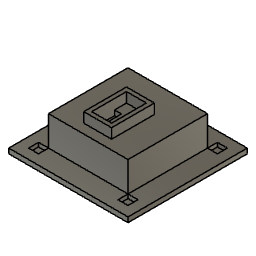
Servo Stand (Autodesk Fusion 360 design; units mm, degrees)
Autodesk Fusion 360 part; units mm, degrees
note: some values were not read from the file. Set by a fixed rule: which face or edge a step refers to.
sketch "Sketch8" plane through (0, 0, 0) normal (0, 0, 1) x (1, 0, 0)
  line L0 (10, 9.5) -> (0, 9.5)
  line L1 (-10, 9.5) -> (0, 9.5)
  line L2 (10, -27.5) -> (-10, -27.5)
  line L3 (-11, 9.5) -> (11.0117, 9.5)
  line L4 (11.0117, 9.5) -> (11.0117, -27.5)
  line L5 (11.0117, -27.5) -> (-11, -27.5)
  line L6 (-11, -27.5) -> (-11, 9.5)
  line L7 (-14, 9.5) -> (-14, 12.5)
  line L8 (-14, 12.5) -> (14, 12.5)
  line L9 (14, 12.5) -> (14, -30.5)
  line L10 (14, -30.5) -> (-14, -30.5)
  line L11 (-14, -30.5) -> (-14, 12.5)
  line L12 (0, 40) -> (-40, 40)
  line L13 (0.0067, -40) -> (40.0067, -39.9933)
  line L14 (-40, 40) -> (40.0067, 40)
  line L15 (40.0067, 40) -> (40.0067, -39.9933)
  line L16 (40.0067, -39.9933) -> (-40, -39.9933)
  line L17 (-40, -39.9933) -> (-40, 40)
  line L18 (-11, -27.5) -> (-11, -17.5)
  line L19 (-11, -17.5) -> (-3, -17.5)
  line L20 (-3, -17.5) -> (-3, -3.5)
  line L21 (-3, -3.5) -> (-11, -3.5)
  line L22 (-11, -3.5) -> (-11, -17.5)
  line L23 (-35, 35) -> (35, 35)
  line L24 (35, 35) -> (35, -35)
  line L25 (35, -35) -> (-35, -35)
  line L26 (-35, -35) -> (-35, 35)
  dimension "d24" = 28
  dimension "d25" = 43
  constraint horizontal L0
  constraint horizontal L1
  constraint horizontal L2
  constraint horizontal L3
  constraint vertical L4
  constraint horizontal L5
  constraint vertical L6
  constraint horizontal L8
  constraint vertical L9
  constraint horizontal L10
  constraint vertical L11
  constraint horizontal L14
  constraint vertical L15
  constraint horizontal L16
  constraint vertical L17
  constraint horizontal L19
  constraint vertical L20
  constraint horizontal L21
  constraint vertical L22
  constraint horizontal L23
  constraint vertical L24
  constraint horizontal L25
  constraint vertical L26
  measures "d24" distance of L7.end L8.end
  measures "d25" distance of L7.end L10.end
extrude "Extrude5" add sketch "Sketch8" against normal blind 30 contours L12 L14 L15 L16 L17 makes body 1
extrude "Extrude6" add sketch "Sketch8" along normal blind 20 separate body contours L7 L8 L9 L10 L11 makes body 2
extrude "Extrude7" add sketch "Sketch8" along normal blind 5 contours L0 L1 L2 L3 L4 L5 L6 L18 L19 L20 L21 | L12 L14 L15 L16 L17 | L23 L24 L25 L26 bodies 1 2
sketch "Sketch9" plane through (-40, 0, 0) normal (-1, 0, 0) x (0, -1, 0)
  line L0 (-40, 5) -> (-40, -30)
  line L1 (-40, -30) -> (39.9933, -30)
  line L2 (39.9933, -30) -> (39.9933, 5)
  line L3 (39.9933, 5) -> (-40, 5)
  line L4 (39.9933, 5) -> (17.4933, 5)
  line L5 (17.4933, 5) -> (17.5013, -6.5)
  line L6 (17.5013, -6.5) -> (3.5013, -6.5)
  line L7 (3.5013, -6.5) -> (3.5013, -13.5)
  line L8 (3.5013, -13.5) -> (17.5013, -13.5)
  line L9 (17.5013, -13.5) -> (17.5013, -6.5)
  dimension "d45" = 22.5
  dimension "d46" = 11.5
  dimension "d47" = 14
  dimension "d48" = 7
  constraint coincident L2.end L3.start
  constraint horizontal L6
  constraint vertical L7
  constraint horizontal L8
  constraint vertical L9
  measures "d45" distance of L2.end L4.end
  measures "d46" distance of L4.end L5.end
  measures "d47" distance of L5.end L6.end
  measures "d48" distance of L5.end L8.end
extrude "Extrude8" cut sketch "Sketch9" against normal blind 14 contours L6 L7 L8 L9 bodies 1
move_body "Move1" bodies 1 to x (1, 0, 0) y (0, 1, 0) z (0, 0, 1) at (0, 0, 30)
sketch "Sketch10" plane through (0, -39.9933, 0) normal (0, -1, 0) x (1, 0, 0)
  line L0 (-40, 35) -> (-40, 0)
  line L1 (-40, 0) -> (40.0067, 0)
  line L2 (40.0067, 0) -> (40.0067, 35)
  line L3 (40.0067, 35) -> (-40, 35)
  line L4 (-40, 0) -> (40.0067, 0)
  line L5 (40.0067, 0) -> (40.0067, 5)
  line L6 (40.0067, 5) -> (-40, 5)
  line L7 (-40, 5) -> (-40, 0)
  dimension "d51" = 80.0067
  dimension "d52" = 5
  constraint horizontal L4
  constraint vertical L5
  constraint horizontal L6
  constraint vertical L7
  constraint coincident L0.end L1.start
  measures "d51" distance of L0.end L1.end
  measures "d52" distance of L0.end L6.end
extrude "Extrude9" add sketch "Sketch10" along normal blind 10 contours L0 L1 L2 L4 L5 L6 L7 bodies 1
sketch "Sketch11" plane through (0, 40, 0) normal (0, 1, 0) x (-1, 0, 0)
  line L0 (-40.0067, 35) -> (-40.0067, 0)
  line L1 (-40.0067, 0) -> (40, 0)
  line L2 (40, 0) -> (40, 35)
  line L3 (40, 35) -> (-40.0067, 35)
  line L4 (-40.0067, 0) -> (40, 0)
  line L5 (40, 0) -> (40, 5)
  line L6 (40, 5) -> (-40.0067, 5)
  line L7 (-40.0067, 5) -> (-40.0067, 0)
  point P0 (40, 5)
  constraint horizontal L4
  constraint vertical L5
  constraint horizontal L6
  constraint vertical L7
  constraint coincident P0 L5.end
  constraint coincident L0.end L1.start
extrude "Extrude10" add sketch "Sketch11" along normal blind 10 contours L0 L1 L2 L4 L5 L6 L7 bodies 1
sketch "Sketch12" plane through (40.0067, 0, 0) normal (1, 0, 0) x (0, 1, 0)
  line L0 (-49.9933, 0) -> (50, 0)
  line L1 (50, 0) -> (50, 5)
  line L2 (50, 5) -> (40, 5)
  line L3 (40, 5) -> (40, 35)
  line L4 (40, 35) -> (-39.9933, 35)
  line L5 (-39.9933, 35) -> (-39.9933, 5)
  line L6 (-39.9933, 5) -> (-49.9933, 5)
  line L7 (-49.9933, 5) -> (-49.9933, 0)
  line L8 (-39.9933, 5) -> (40, 5)
  constraint coincident L5.end L6.start
  constraint coincident L2.end L3.start
extrude "Extrude11" add sketch "Sketch12" along normal blind 10 contours L0 L1 L2 L6 L7 L8 bodies 1
sketch "Sketch13" plane through (-40, 0, 0) normal (-1, 0, 0) x (0, -1, 0)
  line L0 (3.5013, 23.5) -> (17.5013, 23.5)
  line L1 (17.5013, 23.5) -> (17.5013, 16.5)
  line L2 (17.5013, 16.5) -> (3.5013, 16.5)
  line L3 (3.5013, 16.5) -> (3.5013, 23.5)
  line L4 (-50, 0) -> (49.9933, 0)
  line L5 (49.9933, 0) -> (49.9933, 5)
  line L6 (49.9933, 5) -> (39.9933, 5)
  line L7 (39.9933, 5) -> (39.9933, 35)
  line L8 (39.9933, 35) -> (-40, 35)
  line L9 (-40, 35) -> (-40, 5)
  line L10 (-40, 5) -> (-50, 5)
  line L11 (-50, 5) -> (-50, 0)
  line L12 (39.9933, 5) -> (-40, 5)
  constraint coincident L6.end L7.start
  constraint coincident L9.end L10.start
extrude "Extrude12" add sketch "Sketch13" along normal blind 10 contours L4 L5 L6 L10 L11 L12 bodies 1
extrude "Extrude13" add 1 faces at (-16.6644, -49.9933, 3.3333) along direction (0, -1, 0) blind 10 on bodies 1 bodies 1
extrude "Extrude14" add 1 faces at (-50, -23.3288, 1.6667) along direction (-1, 0, 0) blind 10 on bodies 1 bodies 1
extrude "Extrude15" add 1 faces at (50.0067, 13.3356, 3.3333) along direction (1, 0, 0) blind 10 on bodies 1 bodies 1
extrude "Extrude16" add 1 faces at (-19.9978, 50, 1.6667) along direction (0, 1, 0) blind 10 on bodies 1 bodies 1
sketch "Sketch14" plane through (0, 0, 5) normal (0, 0, 1) x (-1, 0, 0)
  line L0 (40, -40) -> (-40.0067, -40)
  line L1 (-40.0067, -40) -> (-40.0067, 39.9933)
  line L2 (-40.0067, 39.9933) -> (40, 39.9933)
  line L3 (40, 39.9933) -> (40, -40)
  line L4 (60, -60) -> (60, 59.9933)
  line L5 (60, 59.9933) -> (-60.0067, 59.9933)
  line L6 (-60.0067, 59.9933) -> (-60.0067, -60)
  line L7 (-60.0067, -60) -> (60, -60)
  line L8 (-40.0067, -40) -> (-50.0067, -40)
  line L9 (-50.0067, -40) -> (-50.0067, -50)
  line L10 (-50.0067, -50) -> (-40.0067, -50)
  line L11 (-40.0067, -50) -> (-40.0067, -40)
  line L12 (40, -40) -> (50, -40)
  line L13 (50, -40) -> (50, -50)
  line L14 (50, -50) -> (40, -50)
  line L15 (40, -50) -> (40, -40)
  line L16 (-40.0067, 39.9933) -> (-50.0067, 39.9933)
  line L17 (-50.0067, 39.9933) -> (-50.0067, 49.9933)
  line L18 (-50.0067, 49.9933) -> (-40.0067, 49.9933)
  line L19 (-40.0067, 49.9933) -> (-40.0067, 39.9933)
  line L20 (40, 39.9933) -> (50, 39.9933)
  line L21 (50, 39.9933) -> (50, 49.9933)
  line L22 (50, 49.9933) -> (40, 49.9933)
  line L23 (40, 49.9933) -> (40, 39.9933)
  dimension "d69" = 10
  dimension "d70" = 10
  dimension "d71" = 10
  dimension "d72" = 10
  dimension "d73" = 10
  dimension "d74" = 10
  dimension "d75" = 10
  constraint horizontal L8
  constraint vertical L9
  constraint horizontal L10
  constraint vertical L11
  constraint coincident L0.end L1.start
  constraint horizontal L12
  constraint vertical L13
  constraint horizontal L14
  constraint vertical L15
  constraint coincident L0.start L3.end
  constraint horizontal L16
  constraint vertical L17
  constraint horizontal L18
  constraint vertical L19
  constraint coincident L1.end L2.start
  constraint horizontal L20
  constraint vertical L21
  constraint horizontal L22
  constraint vertical L23
  constraint coincident L2.end L3.start
  measures "d69" distance of L0.end L8.end
  measures "d70" distance of L0.start L12.end
  measures "d71" distance of L0.start L14.end
  measures "d72" distance of L1.end L16.end
  measures "d73" distance of L1.end L18.end
  measures "d74" distance of L2.end L20.end
  measures "d75" distance of L2.end L22.end
extrude "Extrude17" cut sketch "Sketch14" against normal blind 4 contours L8 L9 L10 L11 | L16 L17 L18 L19 | L20 L21 L22 L23 | L12 L13 L14 L15 bodies 1
extrude "Extrude18" add 1 faces at (3.6744, -27.5, 40) along direction (0, 1, 0) blind 1 on bodies 1 bodies 1
extrude "Extrude19" add 1 faces at (11.0117, -2.5, 40) along direction (-1, 0, 0) blind 1 on bodies 1 bodies 1
extrude "Extrude20" add 1 faces at (-11, -6.8333, 45) along direction (1, 0, 0) blind 1 on bodies 1 bodies 1
extrude "Extrude21" add 2 faces at (3.3333, 9.5, 40) (10.0039, 9.5, 40) along direction (0, -1, 0) blind 1 on bodies 1 bodies 1
extrude "Extrude22" cut 1 faces at (-12.6667, -14.8333, 50) along direction (0, 0, -1) blind 5 on bodies 1 bodies 1
